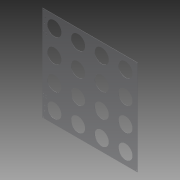
# Autodesk Inventor part: Plastic Funnel PIece
Saved by Autodesk Inventor 2014 (Build 180170000, 170)
## iProperties
Created: 2014-01-04
Part Number: Plastic Funnel PIece
Material: Polycarbonate, Clear
Document SubType Name: Sheet Metal
Designer: Michael
Density: 1.2 g/cm^3
Appearance: Polycarbonate - Clear
Sheet Metal Rule: Default
Author: Michael
Autodesk Inventor part; units mm, degrees
ref_plane "YZ Plane" through (0, 0, 0) normal (1, 0, 0) x (0, 1, 0)
ref_plane "XZ Plane" through (0, 0, 0) normal (0, 1, 0) x (-1, 0, 0)
ref_plane "XY Plane" through (0, 0, 0) normal (0, 0, 1) x (1, 0, 0)
sketch "Sketch1" plane through (0, 0, 0) normal (0, 0, 1) x (1, 0, 0)
  line L0 (0, 0) -> (508, 0)
  line L1 (508, 0) -> (508, 508)
  line L2 (508, 508) -> (0, 508)
  line L3 (0, 508) -> (0, 0)
  line L4 (0, 254) -> (508, 254) construction
  line L5 (254, 508) -> (254, 0) construction
  line L6 (25.4, 482.6) -> (482.6, 482.6) construction
  line L7 (482.6, 482.6) -> (482.6, 25.4) construction
  line L8 (482.6, 25.4) -> (25.4, 25.4) construction
  line L9 (25.4, 25.4) -> (25.4, 482.6) construction
  circle A0 centre (6.35, 501.65) radius 2.4892
  circle A1 centre (501.65, 501.65) radius 2.4892
  circle A2 centre (501.65, 6.35) radius 2.4892
  circle A3 centre (6.35, 6.35) radius 2.4892
  circle A4 centre (6.35, 406.4) radius 2.4892
  circle A5 centre (19.05, 406.4) radius 2.4892
  circle A6 centre (6.35, 393.7) radius 2.4892
  circle A7 centre (19.05, 393.7) radius 2.4892
  circle A8 centre (6.35, 101.6) radius 2.4892
  circle A9 centre (19.05, 101.6) radius 2.4892
  circle A10 centre (6.35, 114.3) radius 2.4892
  circle A11 centre (19.05, 114.3) radius 2.4892
  circle A12 centre (12.7, 469.9) radius 2.4892
  circle A13 centre (12.7, 444.5) radius 2.4892
  circle A14 centre (12.7, 38.1) radius 2.4892
  circle A15 centre (12.7, 63.5) radius 2.4892
  dimension "d5" = 508
  dimension "d6" = 508
  dimension "d12" = 25.4
  dimension "d67" = 4.9784
  dimension "d69" = 6.35
  dimension "d70" = 6.35
  dimension "d82" = 6.35
  dimension "d85" = 12.7
  dimension "d88" = 12.7
  dimension "d91" = 101.6
  dimension "d92" = 4.9784
  dimension "d93" = 12.7
  dimension "d94" = 38.1
  dimension "d97" = 25.4
  constraints: 20 end point, 16 centre point, 9 symmetric about line, 4 midpoint, 4 parallel, 2 horizontal, 2 perpendicular, 2 vertical, 1 equal radius, 20 other
  measures "d5" distance of L2.end L1.end
  measures "d6" distance of L1.end L0.end
  measures "d12" distance between parallel lines of L6 L2
  measures "d67" diameter of A0
  measures "d69" distance from line of L2 A0.centre
  measures "d70" distance from line of L3 A0.centre
  measures "d82" distance from line of L3 A4.centre
  measures "d85" distance of A4.centre A5.centre
  measures "d88" distance of A4.centre A6.centre
  measures "d91" distance from line of L2 A4.centre
  measures "d92" diameter of A12
  measures "d93" distance from line of L3 A12.centre
  measures "d94" distance from line of L2 A12.centre
  measures "d97" distance of A12.centre A13.centre
extrude "Extrusion1" add sketch "Sketch1" along normal blind 1.5875
sketch "Sketch3" plane through (0, 0, 0) normal (0, 0, -1) x (-1, 0, 0)
  line L0 (-508, 508) -> (0, 508) projected
  line L1 (-508, 0) -> (-508, 508) projected
  circle A0 centre (-444.5, 444.5) radius 38.1
  dimension "d26" = 76.2
  dimension "d27" = 63.5
  dimension "d28" = 63.5
  constraints: 1 centre point
  measures "d26" diameter of A0
  measures "d27" distance from line of L0 A0.centre
  measures "d28" distance from line of L1 A0.centre
extrude "Extrusion3" cut sketch "Sketch3" against normal blind 1.5875
pattern_linear "Rectangular Pattern1" count 4 spacing 127 along (-1, 0, 0) count 4 spacing 127 along (0, -1, 0) of "Extrusion3"
equation "\"BendRadius\" = Thickness"
equation "\"BendReliefWidth\" = Thickness"
equation "\"BendReliefDepth\" = 0.5 * Thickness"
equation "\"CornerReliefSize\" = 4 * Thickness"
equation "\"MinimumRemnant\" = 2 * Thickness"
equation "\"TransitionRadius\" = BendRadius"
equation "\"JacobiRadiusSize\" = Thickness"
equation "\"GapSize\" = Thickness"
equation "\"Thickness\" = 3.048"
body "Solid2"
